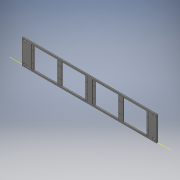
# Autodesk Inventor part: Ra-Manager_Painel_Frontal
Saved by Autodesk Inventor 2019 (Build 230136000, 136)
## iProperties
Created: 2020-03-06
Part Number: Ra-Manager_Painel_Frontal
Material: Aço, carbono
Document SubType Name: Modeling
Designer: caio.santos
Density: 7.85 g/cm^3
Appearance: Semipolido
Author: caio.santos
Autodesk Inventor part; units mm, degrees
ref_plane "YZ Plane" through (0, 0, 0) normal (1, 0, 0) x (0, 1, 0)
ref_plane "XZ Plane" through (0, 0, 0) normal (0, 1, 0) x (-1, 0, 0)
ref_plane "XY Plane" through (0, 0, 0) normal (0, 0, 1) x (1, 0, 0)
sketch "Esboço1" plane through (0, 0, 0) normal (0, 0, 1) x (1, 0, 0)
  line L0 (-241.25, 44) -> (241.25, 44)
  line L1 (241.25, 44) -> (241.25, -44)
  line L2 (241.25, -44) -> (-241.25, -44)
  line L3 (-241.25, -44) -> (-241.25, 44)
  point P0 (0, 0)
  dimension "d0" = 482.5
  dimension "d1" = 88
  dimension "d2" = 44
  dimension "d3" = 241.25
  constraints: 8 end point, 2 parallel, 1 horizontal, 1 perpendicular
  measures "d0" distance of L0.start L0.end
  measures "d1" distance of L2.end L0.start
  measures "d2" distance from line of point (0, 0) L0
  measures "d3" distance from line of point (0, 0) L3
extrude "Extrusão1" add sketch "Esboço1" along normal blind 4
sketch "Esboço2" plane through (0, 0, 4) normal (0, 0, 1) x (1, 0, 0)
  line L0 (237.7245, 44) -> (-241.25, 44)
  line L1 (-241.25, 44) -> (-241.25, 0.6073)
  line L2 (-235.5, 41) -> (-230, 41)
  line L3 (-226.75, 41.6246) -> (-226.75, 34.6246)
  line L4 (-226.75, 34.6246) -> (-238.75, 34.6246)
  line L5 (-238.75, 34.6246) -> (-238.75, 40.8421)
  arc A0 (-235.5, 41) -> (-235.5, 34.6246) centre (-235.5617, 37.8123) ccw
  arc A1 (-230, 34.6246) -> (-230, 41) centre (-229.9383, 37.8123) ccw
  line L6 (-230, 41) -> (-230, 34.6246) construction
  line L7 (-230, 41) -> (-223.6246, 41) construction
  line L8 (241.25, 44) -> (-241.25, 44) projected
  line L9 (-241.25, 44) -> (-241.25, -44) projected
  point P0 (0, 0)
  dimension "d6" = 7
  dimension "d7" = 12
  dimension "d8" = 2.5
  dimension "d9" = 3
  dimension "d10" = 90
  dimension "d11" = 5.5
  dimension "d12" = 3.1883
  dimension "d13" = 3.1883
  dimension "d14" = 0
  dimension "d15" = 0
  constraints: 16 end point, 4 point on circle, 2 centre point, 2 horizontal, 2 parallel, 2 perpendicular, 2 point on line, 2 tangent, 1 horizontal alignment
  measures "d6" distance of L3.start L3.end
  measures "d7" distance of L3.end L4.end
  measures "d8" distance between parallel lines of L5 L1
  measures "d9" distance between parallel lines of L0 L2
  measures "d10" angle of L6 L7
  measures "d11" distance of L2.start L2.end
  measures "d12" distance from line of L5 A0.centre
  measures "d13" distance from line of L3 A1.centre
  measures "d14" distance between parallel lines of L8 L0
  measures "d15" distance between parallel lines of L9 L1
extrude "Extrusão2" cut sketch "Esboço2" against normal blind 10 contours L2 A1 L4 A0
pattern_linear "Padrão retangular1" count 2 spacing 73 along (0, -1, 0) count 2 spacing 465.5 along (1, 0, 0) of "Extrusão2"
sketch "Esboço5" plane through (0, 0, 4) normal (0, 0, 1) x (1, 0, 0)
  line L0 (0, 44) -> (0, -44) construction
  line L1 (-215, -44) -> (217, -44) construction
  line L2 (217, -44) -> (217, 44) construction
  line L3 (-213, -39) -> (217, -39) construction
  line L4 (-202, 39) -> (-202, -39)
  line L5 (-202, 39) -> (-117, 39)
  line L6 (-117, 39) -> (-117, -39)
  line L7 (-202, -39) -> (-117, -39)
  line L8 (-241.25, 44) -> (-241.25, -44) projected
  line L9 (241.25, 44) -> (-241.25, 44) projected
  line L10 (-101, 39) -> (-16, 39)
  line L11 (-101, 39) -> (-101, -39)
  line L12 (-16, 39) -> (-16, -39)
  line L13 (-101, -39) -> (-16, -39)
  line L14 (-117, 19.5) -> (-101, 19.5) construction
  line L15 (-241.25, 19.5) -> (241.25, 19.5) construction
  line L16 (241.25, -44) -> (241.25, 44) projected
  line L17 (-242, -19.5) -> (241.25, -19.5) construction
  line L18 (-215, 44) -> (-215, -44) construction
  line L19 (-241.25, -44) -> (241.25, -44) projected
  line L20 (204, 39) -> (204, -39)
  line L21 (204, 39) -> (119, 39)
  line L22 (119, 39) -> (119, -39)
  line L23 (204, -39) -> (119, -39)
  line L24 (119, 39) -> (103, 39)
  line L25 (103, 39) -> (103, -39)
  line L26 (119, -39) -> (103, -39)
  line L27 (103, 39) -> (18, 39)
  line L28 (18, 39) -> (18, -39)
  line L29 (103, -39) -> (18, -39)
  line L30 (18, -39) -> (10, -39)
  line L31 (10, 39) -> (18, 39)
  line L32 (-16, 39) -> (-8, 39)
  line L33 (-8, 39) -> (-8, -39)
  line L34 (-16, -39) -> (-8, -39)
  line L35 (10, 39) -> (10, -39)
  line L36 (111, 39) -> (111, -39) construction
  line L37 (-117, 39) -> (-101, 39)
  line L38 (-101, -39) -> (-117, -39)
  line L39 (212, 39) -> (212, -39)
  line L40 (212, 39) -> (204, 39)
  line L41 (212, -39) -> (204, -39)
  line L42 (-210, 39) -> (-210, -39)
  line L43 (-210, 39) -> (-202, 39)
  line L44 (-210, -39) -> (-202, -39)
  line L45 (-109, 44) -> (-109, -44) construction
  line L46 (241.25, -44) -> (-241.25, -44) projected
  point P0 (0, 0)
  dimension "d58" = 430
  dimension "d68" = 5
  dimension "d69" = 5
  dimension "d73" = 101
  dimension "d79" = 85
  dimension "d84" = 85
  dimension "d85" = 16
  dimension "d86" = 85
  dimension "d87" = 8
  dimension "d88" = 8
  dimension "d89" = 88
  dimension "d90" = 456.25
  dimension "d91" = 24.5
  dimension "d92" = 63.5
  dimension "d93" = 24.5
  dimension "d94" = 241.25
  dimension "d95" = 0
  dimension "d96" = 88
  dimension "d97" = 483.25
  dimension "d140" = 5
  dimension "d141" = 78
  dimension "d142" = 451.25
  dimension "d209" = 90
  dimension "d210" = 90
  dimension "d211" = 90
  dimension "d212" = 90
  dimension "d213" = 90
  dimension "d214" = 5
  dimension "d215" = 458.25
  constraints: 82 end point, 9 horizontal, 9 point on line, 9 vertical, 6 perpendicular, 4 collinear, 2 midpoint, 2 parallel, 18 other
  measures "d58" distance of point (-213, -39) point (217, -39)
  measures "d68" distance between parallel lines of L1 L7
  measures "d69" distance between parallel lines of L9 L5
  measures "d73" distance of L4.start L10.start
  measures "d79" distance of L4.end L6.end
  measures "d84" distance of L20.start L21.end
  measures "d85" distance of L21.end L24.end
  measures "d86" distance of L24.end L27.end
  measures "d87" distance of L10.end L32.end
  measures "d88" distance of L31.start L27.end
  measures "d89" distance of L1.end L2.end
  measures "d90" distance between parallel lines of L16 L18
  measures "d91" distance between parallel lines of L15 L9
  measures "d92" distance between parallel lines of L17 L9
  measures "d93" distance between parallel lines of L14 L9
  measures "d94" distance between parallel lines of L0 L16
  measures "d95" distance from line of L0.start L9
  measures "d96" distance from line of L0.end L9
  measures "d97" distance from line of L17.start L16
  measures "d140" distance between parallel lines of L2 L39
  measures "d141" distance of L42.start L42.end
  measures "d142" distance between parallel lines of L16 L42
  measures "d209" angle of L8 L24
  measures "d210" angle of L8 L31
  measures "d211" angle of L8 L43
  measures "d212" angle of L21 L16
  measures "d213" angle of L32 L16
  measures "d214" distance between parallel lines of L9 L40
  measures "d215" distance between parallel lines of L8 L2
extrude "Extrusão8" cut sketch "Esboço5" against normal blind 2 contours L4 L44 L42 L43 | L37 L11 L38 L6 | L32 L33 L34 L12 | L40 L39 L41 L20 | L22 L26 L25 L24 | L28 L30 L35 L31
sketch "Esboço9" plane through (0, 0, 4) normal (0, 0, 1) x (1, 0, 0)
  line L0 (0, 44) -> (0, -44) construction
  line L1 (-215, -44) -> (217, -44) construction
  line L2 (217, -44) -> (217, 44) construction
  line L3 (-213, -39) -> (217, -39) construction
  line L4 (-202, 39) -> (-202, -39)
  line L5 (-202, 39) -> (-117, 39)
  line L6 (-117, 39) -> (-117, -39)
  line L7 (-202, -39) -> (-117, -39)
  line L8 (-241.25, 44) -> (-241.25, -44)
  line L9 (241.25, 44) -> (-241.25, 44)
  line L10 (-101, 39) -> (-16, 39)
  line L11 (-101, 39) -> (-101, -39)
  line L12 (-16, 39) -> (-16, -39)
  line L13 (-101, -39) -> (-16, -39)
  line L14 (-117, 19.5) -> (-101, 19.5) construction
  line L15 (-241.25, 19.5) -> (241.25, 19.5) construction
  line L16 (241.25, -44) -> (241.25, 44)
  line L17 (-242, -19.5) -> (241.25, -19.5) construction
  line L18 (-215, 44) -> (-215, -44) construction
  line L19 (-241.25, -44) -> (241.25, -44)
  line L20 (204, 39) -> (204, -39)
  line L21 (204, 39) -> (119, 39)
  line L22 (119, 39) -> (119, -39)
  line L23 (204, -39) -> (119, -39)
  line L24 (119, 39) -> (103, 39)
  line L25 (103, 39) -> (103, -39)
  line L26 (119, -39) -> (103, -39)
  line L27 (103, 39) -> (18, 39)
  line L28 (18, 39) -> (18, -39)
  line L29 (103, -39) -> (18, -39)
  line L30 (18, -39) -> (10, -39)
  line L31 (10, 39) -> (18, 39)
  line L32 (-16, 39) -> (-8, 39)
  line L33 (-8, 39) -> (-8, -39)
  line L34 (-16, -39) -> (-8, -39)
  line L35 (10, 39) -> (10, -39)
  line L36 (111, 39) -> (111, -39) construction
  line L37 (-117, 39) -> (-101, 39)
  line L38 (-101, -39) -> (-117, -39)
  line L39 (212, 39) -> (212, -39)
  line L40 (212, 39) -> (204, 39)
  line L41 (212, -39) -> (204, -39)
  line L42 (-210, 39) -> (-210, -39)
  line L43 (-210, 39) -> (-202, 39)
  line L44 (-210, -39) -> (-202, -39)
  line L45 (-109, 44) -> (-109, -44) construction
  line L46 (241.25, -44) -> (-241.25, -44)
  point P0 (0, 0)
  point P1 (0, 0)
  dimension "d222" = 430
  dimension "d223" = 5
  dimension "d224" = 5
  dimension "d225" = 101
  dimension "d226" = 85
  dimension "d227" = 85
  dimension "d228" = 16
  dimension "d229" = 85
  dimension "d230" = 8
  dimension "d231" = 8
  dimension "d232" = 88
  dimension "d233" = 456.25
  dimension "d234" = 24.5
  dimension "d235" = 63.5
  dimension "d236" = 24.5
  dimension "d237" = 241.25
  dimension "d238" = 0
  dimension "d239" = 88
  dimension "d240" = 483.25
  dimension "d241" = 5
  dimension "d242" = 78
  dimension "d243" = 451.25
  dimension "d244" = 90
  dimension "d245" = 90
  dimension "d246" = 90
  dimension "d247" = 90
  dimension "d248" = 90
  dimension "d249" = 5
  dimension "d250" = 458.25
  dimension "d252" = 88
  dimension "d253" = 24.25
  dimension "d254" = 350.25
  dimension "d255" = 44
  dimension "d256" = 241.25
  dimension "d257" = 44
  dimension "d258" = 241.25
  constraints: 92 end point, 9 horizontal, 9 point on line, 9 vertical, 6 perpendicular, 4 collinear, 2 midpoint, 2 parallel, 18 other
  measures "d222" distance of point (-213, -39) point (217, -39)
  measures "d223" distance between parallel lines of L1 L7
  measures "d224" distance between parallel lines of L9 L5
  measures "d225" distance of L4.start L10.start
  measures "d226" distance of L4.end L6.end
  measures "d227" distance of L20.start L21.end
  measures "d228" distance of L21.end L24.end
  measures "d229" distance of L24.end L27.end
  measures "d230" distance of L10.end L32.end
  measures "d231" distance of L31.start L27.end
  measures "d232" distance of L1.end L2.end
  measures "d233" distance between parallel lines of L16 L18
  measures "d234" distance between parallel lines of L15 L9
  measures "d235" distance between parallel lines of L17 L9
  measures "d236" distance between parallel lines of L14 L9
  measures "d237" distance between parallel lines of L0 L16
  measures "d238" distance from line of L0.start L9
  measures "d239" distance from line of L0.end L9
  measures "d240" distance from line of L17.start L16
  measures "d241" distance between parallel lines of L2 L39
  measures "d242" distance of L42.start L42.end
  measures "d243" distance between parallel lines of L16 L42
  measures "d244" angle of L8 L24
  measures "d245" angle of L8 L31
  measures "d246" angle of L8 L43
  measures "d247" angle of L21 L16
  measures "d248" angle of L32 L16
  measures "d249" distance between parallel lines of L9 L40
  measures "d250" distance between parallel lines of L8 L2
  measures "d252" distance between parallel lines of L46 L9
  measures "d253" distance between parallel lines of L2 L16
  measures "d254" distance between parallel lines of L45 L16
  measures "d255" distance from line of point (0, 0) L9
  measures "d256" distance from line of point (0, 0) L16
  measures "d257" distance from line of point (0, 0) L9
  measures "d258" distance from line of point (0, 0) L16
extrude "Extrusão9" cut sketch "Esboço9" against normal blind 10 contours L5 L6 L7 L4 | L10 L12 L13 L11 | L20 L23 L22 L21 | L25 L29 L28 L27
sketch "Esboço10" plane through (0, 0, 2) normal (0, 0, 1) x (1, 0, 0)
  line L0 (-117, -39) -> (-117, 39) projected
  line L1 (-210, -39) -> (-210, 39) projected
  line L2 (-210, 19.5) -> (212, 19.5) construction
  line L3 (-210, -19.5) -> (212, -19.5) construction
  line L4 (212, 39) -> (212, -39) projected
  line L5 (-206, 39) -> (-206, -39) construction
  line L6 (-117, 39) -> (-101, 39) projected
  line L7 (-109, 39) -> (-109, -39)
  line L8 (-113, 39) -> (-113, -39) construction
  line L9 (-105, 39) -> (-105, -39) construction
  line L10 (-241.25, -44) -> (241.25, -44) projected
  line L11 (-8, -39) -> (-210, -39) projected
  line L12 (-12, -39) -> (-12, 39) construction
  line L13 (14, 39) -> (14, -39) construction
  line L14 (103, 39) -> (119, 39) projected
  line L15 (111, 39) -> (111, -39)
  line L16 (107, 39) -> (107, -39) construction
  line L17 (119, -39) -> (103, -39) projected
  line L18 (115, -39) -> (115, 39) construction
  line L19 (208, 39) -> (208, -39) construction
  point P0 (0, 0)
  point P1 (-206, 19.5)
  point P2 (-206, -19.5)
  point P3 (-113, 19.5)
  point P4 (-105, 19.5)
  point P5 (-105, -19.5)
  point P6 (-113, -19.5)
  point P7 (-12, -19.5)
  point P8 (-12, 19.5)
  point P9 (14, 19.5)
  point P10 (14, -19.5)
  point P11 (107, 19.5)
  point P12 (115, 19.5)
  point P13 (115, -19.5)
  point P14 (107, -19.5)
  point P15 (208, -19.5)
  point P16 (208, 19.5)
  dimension "d263" = 4
  dimension "d264" = 97
  dimension "d265" = 105
  dimension "d266" = 198
  dimension "d267" = 224
  dimension "d268" = 317
  dimension "d269" = 325
  dimension "d270" = 418
  dimension "d271" = 58.5
  dimension "d272" = 19.5
  dimension "d273" = 0
  dimension "d274" = 78
  dimension "d275" = 0
  dimension "d276" = 0
  dimension "d277" = 78
  dimension "d278" = 0
  dimension "d279" = 78
  dimension "d280" = 0
  dimension "d281" = 0
  dimension "d282" = 0
  dimension "d283" = 78
  dimension "d284" = 0
  constraints: 26 point on line, 20 end point, 6 vertical, 3 perpendicular, 2 midpoint, 1 parallel, 22 other
  measures "d263" distance between parallel lines of L4 L19
  measures "d264" distance between parallel lines of L4 L18
  measures "d265" distance between parallel lines of L4 L16
  measures "d266" distance between parallel lines of L4 L13
  measures "d267" distance between parallel lines of L4 L12
  measures "d268" distance between parallel lines of L4 L9
  measures "d269" distance between parallel lines of L4 L8
  measures "d270" distance between parallel lines of L4 L5
  measures "d273" distance from line of point (212, 19.5) L4
  measures "d274" distance from line of L19.start L17
  measures "d275" distance from line of L19.end L17
  measures "d276" distance from line of L15.end L17
  measures "d277" distance from line of L13.start L17
  measures "d278" distance from line of L13.end L17
  measures "d279" distance from line of L12.end L17
  measures "d280" distance from line of L9.end L17
  measures "d281" distance from line of L7.end L17
  measures "d282" distance from line of L8.end L17
  measures "d283" distance from line of L5.start L17
  measures "d284" distance from line of L5.end L17
hole "Furo2" at (-206, 19.5, 2) at (-206, -19.5, 2) at (-113, 19.5, 2) at (-105, 19.5, 2) at (-105, -19.5, 2) at (-113, -19.5, 2) at (-12, -19.5, 2) at (-12, 19.5, 2) at (14, 19.5, 2) at (14, -19.5, 2) at (107, 19.5, 2) at (115, 19.5, 2) at (115, -19.5, 2) at (107, -19.5, 2) at (208, -19.5, 2) at (208, 19.5, 2) direction (0, 0, -1) diameter 2.459 end through all thread size "M3x0.5" class "6H" standard "ANSI Metric M Profile"
equation "\"d2\" = 0.5 * d1"
equation "\"d3\" = 0.5 * d0"
equation "\"d12\" = d13"
